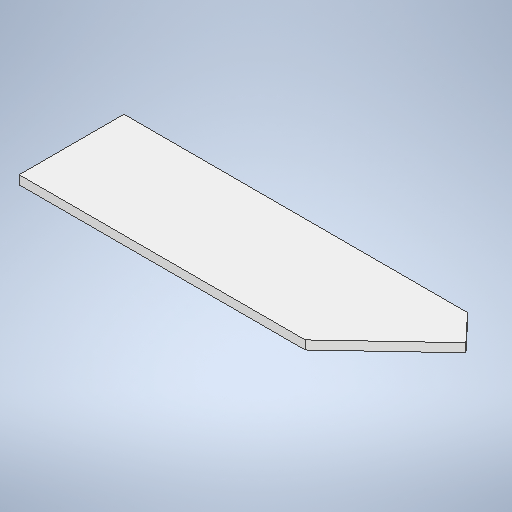
# Autodesk Inventor part: Quartz_Countertop--1.5_x_18_x_63.34829
Saved by Autodesk Inventor 2025 (Build 290162000, 162)
## iProperties
Created: 2023-05-06
Part Number: Quartz_Countertop--1.5_x_18_x_63.34829
Material: Generic
Document SubType Name: Modeling
Designer: Tom
Density: 1 g/cm^3
Appearance: White
Author: Tom
Autodesk Inventor part; units mm, degrees
ref_plane "YZ Plane" through (0, 0, 0) normal (1, 0, 0) x (0, 1, 0)
ref_plane "XZ Plane" through (0, 0, 0) normal (0, 1, 0) x (-1, 0, 0)
ref_plane "XY Plane" through (0, 0, 0) normal (0, 0, 1) x (1, 0, 0)
sketch "Sketch1" plane through (0, 0, 0) normal (0, 1, 0) x (-1, 0, 0)
  line L0 (0, 0) -> (-1609.0466, 0)
  line L1 (-1609.0466, 0) -> (-1609.0466, -457.2)
  line L2 (-1609.0466, -457.2) -> (0, -457.2)
  line L3 (0, -457.2) -> (0, 0)
  dimension "d6" = 457.2
  dimension "d10" = 1609.0466
  constraints: 8 end point, 2 parallel, 1 coincident, 1 horizontal, 1 perpendicular
  measures "d6" distance of L2.end L0.start
  measures "d10" distance of L1.end L2.end
extrude "Extrusion1" add sketch "Sketch1" along normal blind 38.1
sketch "Sketch3" plane through (0, 38.1, 0) normal (0, 1, 0) x (1, 0, 0)
  line L0 (1609.0466, 457.2) -> (0, 457.2) projected
  line L1 (1498.5999, 457.2) -> (1609.0466, 339.8328)
  line L2 (1609.0466, 0) -> (1609.0466, 457.2) projected
  line L3 (1609.0466, 339.8328) -> (1247.9199, 0)
  line L4 (0, 0) -> (1609.0466, 0) projected
  dimension "d16" = 133.26
  dimension "d17" = 161.163
  constraints: 4 end point, 3 point on line, 1 perpendicular
  measures "d16" angle of L1 L0
  measures "d17" distance of L1.start L1.end
extrude "Extrusion3" cut sketch "Sketch3" against normal up to surface (38.1 mm away)
body "Solid1"
